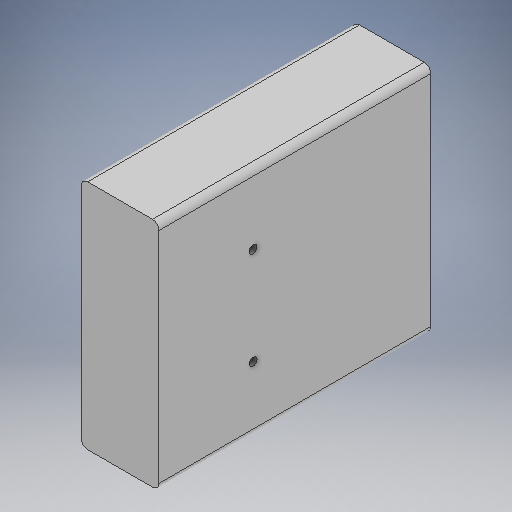
# Autodesk Inventor part: Meinberg_Box
Saved by Autodesk Inventor 2025.3 (Build 293356000, 356)
## iProperties
Created: 2025-12-17
Part Number: Meinberg_Box
Material: Generic
Document SubType Name: Modeling
Designer: sonata
Density: 1 g/cm^3
Appearance: Default
Author: sonata
Autodesk Inventor part; units mm, degrees
ref_plane "YZ Plane" through (0, 0, 0) normal (1, 0, 0) x (0, 1, 0)
ref_plane "XZ Plane" through (0, 0, 0) normal (0, 1, 0) x (-1, 0, 0)
ref_plane "XY Plane" through (0, 0, 0) normal (0, 0, 1) x (1, 0, 0)
sketch "Sketch1" plane through (0, 0, 0) normal (1, 0, 0) x (0, 1, 0)
  line L0 (0, 0) -> (71.5, 0)
  line L1 (71.5, 0) -> (71.5, -83.8)
  line L2 (71.5, -83.8) -> (0, -83.8)
  line L3 (0, -83.8) -> (0, 0)
  dimension "d0" = 83.8
  dimension "d1" = 71.5
  constraints: 8 end point, 2 parallel, 1 horizontal, 1 perpendicular
  measures "d0" distance of L0.end L1.end
  measures "d1" distance of L1.end L2.end
extrude "Extrusion1" add sketch "Sketch1" along normal blind 24
fillet "Fillet1" radius 2 4 edges at (24, 71.5, -41.9) (0, 71.5, -41.9) (24, 0, -41.9) (0, 0, -41.9)
sketch "Sketch4" plane through (24, 0, 0) normal (1, 0, 0) x (0, 0, -1)
  line L0 (0, 0) -> (83.8, 0) projected
  line L1 (0, 69.5) -> (0, 2) projected
  point P0 (29, 20)
  point P1 (29, 50)
  dimension "d22" = 20
  dimension "d23" = 50
  dimension "d24" = 29
  constraints: 1 vertical alignment
  measures "d22" distance from line of point (29, 20) L0
  measures "d23" distance from line of L0 point (29, 50)
  measures "d24" distance from line of L1 point (29, 20)
hole "Hole3" at (24, 20, -29) at (24, 50, -29) direction (-1, 0, 0) diameter 2.459 depth 6 thread size "M3x0.5" class "6H" standard "ANSI Metric M Profile"
body "Solid1"
